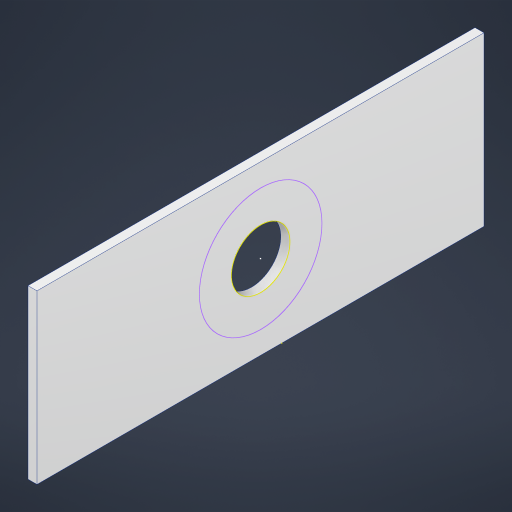
# Autodesk Inventor part: Osnova
Saved by Autodesk Inventor 2024 (Build 280153000, 153)
## iProperties
Created: 2023-12-23
Part Number: Osnova
Material: Aluminum 6061
Document SubType Name: Modeling
Designer: KirikDK
Mass: 2401.32 g
Surface Area: 1935.57 cm^2
Volume: 889.377 cm^3
Density: 2.7 g/cm^3
Appearance: Aluminum - Flat
Author: KirikDK
Autodesk Inventor part; units mm, degrees
ref_plane "YZ Plane" through (0, 0, 0) normal (1, 0, 0) x (0, 1, 0)
ref_plane "XZ Plane" through (0, 0, 0) normal (0, 1, 0) x (-1, 0, 0)
ref_plane "XY Plane" through (0, 0, 0) normal (0, 0, 1) x (1, 0, 0)
sketch "Sketch1" plane through (0, 0, 0) normal (0, 1, 0) x (-1, 0, 0)
  line L0 (95, 271.4286) -> (85, 271.4286)
  line L1 (85, 271.4286) -> (85, -224.5714)
  line L2 (85, -224.5714) -> (95, -224.5714)
  line L3 (95, -224.5714) -> (95, 271.4286)
  point P0 (0, 0)
  dimension "d0" = 10
  dimension "d1" = 496
  constraints: 8 end point, 2 parallel, 1 horizontal, 1 perpendicular
  measures "d0" distance of L0.start L0.end
  measures "d1" distance of L2.end L0.start
extrude "Extrusion1" add sketch "Sketch1" along normal blind 186
sketch "Sketch3" plane through (-85, 0, 271.4286) normal (1, 0, 0) x (0, 0, -1)
  line L0 (0, 0) -> (496, 0) projected
  line L1 (496, 0) -> (496, 186) projected
  line L2 (0, 186) -> (496, 186) projected
  line L3 (0, 0) -> (0, 186) projected
  circle A0 centre (0, 93) radius 5
  line L4 (0, 0) -> (496, 0) projected
  circle A1 centre (248, 0) radius 5
  line L5 (0, 0) -> (248, 0)
  line L6 (0, 93) -> (0, 0)
  circle A2 centre (248, 93) radius 32.5
  point P0 (271.4286, 0)
  dimension "d16" = 65
  dimension "d19" = 93
  dimension "d20" = 248
  dimension "d21" = 248
  dimension "d22" = 93
  constraints: 4 end point, 3 centre point, 3 midpoint, 1 horizontal
  measures "d16" diameter of A2
  measures "d19" distance of point (248, 0) A2.centre
  measures "d20" distance from line of L3 A2.centre
  measures "d21" distance from line of L1 A2.centre
  measures "d22" distance from line of L2 A2.centre
extrude "Extrusion5" cut sketch "Sketch3" against normal blind 186 contours A2
sketch "Sketch4" plane through (-85, 0, 271.4286) normal (1, 0, 0) x (0, 0, -1)
  circle A0 centre (248, 93) radius 32.5 projected
  circle A1 centre (248, 93) radius 68
  point P0 (271.4286, 0)
  constraints: 1 centre point, 1 coincident
body "Solid1"
